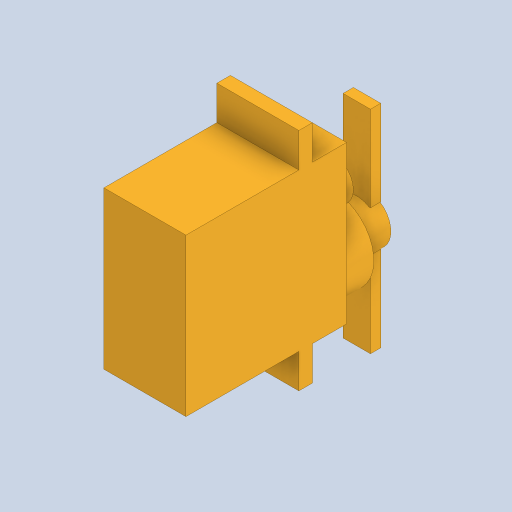
# Autodesk Inventor part: Servo
Saved by Autodesk Inventor 2023.1 (Build 271208000, 208)
## iProperties
Created: 2024-08-02
Part Number: Servo
Material: S355J2+N
Document SubType Name: Modeling
Designer: huchonms
Engineer: thingelstade
Mass: 59.7282 g
Surface Area: 30.452 cm^2
Volume: 7.60868 cm^3
Density: 7.85 g/cm^3
Appearance: Metal (300-500 MPa)
tc_part_rev_length: 12
tc_part_rev_width: 32.5
tc_part_rev_height: 37.54
tc_part_rev_uom_length: mm
tc_part_rev_volume: 7609
tc_part_rev_uom_volume: mm^3
tc_part_rev_mass: 0.06
tc_part_rev_uom_mass: kg
NOV_FileName: Servo
Author: huchonms
Revision Number: 0
Autodesk Inventor part; units mm, degrees
ref_plane "YZ Plane" through (0, 0, 0) normal (1, 0, 0) x (0, 1, 0)
ref_plane "XZ Plane" through (0, 0, 0) normal (0, 1, 0) x (-1, 0, 0)
ref_plane "XY Plane" through (0, 0, 0) normal (0, 0, 1) x (1, 0, 0)
sketch "Sketch1" plane through (0, 0, 0) normal (0, 1, 0) x (-1, 0, 0)
  line L0 (-6, -11.5) -> (6, -11.5)
  line L1 (6, -11.5) -> (6, 11.5)
  line L2 (6, 11.5) -> (-6, 11.5)
  line L3 (-6, 11.5) -> (-6, -11.5)
  line L4 (-6, -11.5) -> (6, 11.5) construction
  line L5 (6, -11.5) -> (-6, 11.5) construction
  point P0 (0, 0)
  dimension "d0" = 12
  dimension "d1" = 23
  constraints: 12 end point, 2 midpoint, 2 parallel, 1 horizontal, 1 perpendicular
  measures "d0" distance of L2.end L1.end
  measures "d1" distance of L1.end L0.end
extrude "Extrusion1" add sketch "Sketch1" along normal blind 23.5
sketch "Sketch2" plane through (-6, 0, -11.5) normal (-1, 0, 0) x (0, 0, 1)
  line L0 (0, 23.5) -> (23, 23.5) projected
  line L1 (0, 18.5) -> (23, 18.5)
  line L2 (0, 18.5) -> (0, 16.523)
  line L3 (0, 16.523) -> (23, 16.523)
  line L4 (23, 16.523) -> (23, 18.5)
  point P0 (11.5, 0)
  dimension "d7" = 5
  constraints: 8 end point, 2 perpendicular, 1 horizontal, 1 vertical
  measures "d7" distance between parallel lines of L1 L0
extrude "Extrusion2" add sketch "Sketch2" along normal blind 5
sketch "Sketch3" plane through (6, 0, 11.5) normal (1, 0, 0) x (0, 0, -1)
  line L0 (0, 16.523) -> (0, 18.5) projected
  line L1 (0, 18.5) -> (23, 18.5) projected
  line L2 (23, 18.5) -> (23, 16.523) projected
  line L3 (23, 16.523) -> (0, 16.523) projected
  point P0 (11.5, 0)
extrude "Extrusion3" add sketch "Sketch3" along normal blind 5
sketch "Sketch4" plane through (0, 23.5, 0) normal (0, 1, 0) x (1, 0, 0)
  circle A0 centre (0, 5.5) radius 6
  line L0 (6, 11.5) -> (-6, 11.5) projected
  point P0 (0, 0)
  dimension "d12" = 12
  dimension "d13" = 6
  constraints: 1 centre point
  measures "d12" diameter of A0
  measures "d13" distance from line of L0 A0.centre
extrude "Extrusion4" add sketch "Sketch4" along normal blind 4
sketch "Sketch6" plane through (0, 23.5, 0) normal (0, 1, 0) x (1, 0, 0)
  circle A0 centre (0, -2) radius 3
  point P0 (0, 0)
  dimension "d17" = 6
  constraints: 1 centre point
  measures "d17" diameter of A0
extrude "Extrusion5" add sketch "Sketch6" along normal up to surface (4 mm away)
sketch "Sketch7" plane through (-6, 0, 11.5) normal (0, 0, 1) x (1, 0, 0)
  line L0 (12, 18.5) -> (17, 18.5) projected
  line L1 (0, 18.5) -> (-5, 18.5) projected
  line L2 (0, 16.523) -> (-5, 16.523) projected
  line L3 (12, 16.523) -> (17, 16.523) projected
  line L4 (0, 18.5) -> (0, 16.523)
  line L5 (0, 16.523) -> (12, 16.523)
  line L6 (12, 16.523) -> (12, 18.5)
  line L7 (0, 18.5) -> (12, 18.5)
  point P0 (6, 0)
  constraints: 8 end point, 2 perpendicular, 1 horizontal, 1 vertical
extrude "Extrusion6" add sketch "Sketch7" along normal blind 5
sketch "Sketch8" plane through (6, 0, -11.5) normal (0, 0, -1) x (-1, 0, 0)
  line L0 (0, 18.5) -> (12, 18.5) projected
  line L1 (12, 18.5) -> (12, 16.523) projected
  line L2 (12, 16.523) -> (0, 16.523) projected
  line L3 (0, 16.523) -> (0, 18.5) projected
  point P0 (6, 0)
extrude "Extrusion7" add sketch "Sketch8" along normal blind 5
sketch "Sketch9" plane through (11, 0, 11.5) normal (1, 0, 0) x (0, 0, -1)
  line L0 (23, 16.523) -> (23, 18.5) projected
  line L1 (23, 18.5) -> (0, 18.5) projected
  line L2 (0, 18.5) -> (0, 16.523) projected
  line L3 (0, 16.523) -> (23, 16.523) projected
  point P0 (11.5, 0)
extrude "Extrusion8" cut sketch "Sketch9" against normal up to surface (5 mm away)
sketch "Sketch10" plane through (-11, 0, -11.5) normal (-1, 0, 0) x (0, 0, 1)
  line L0 (23, 16.523) -> (23, 18.5) projected
  line L1 (23, 18.5) -> (0, 18.5) projected
  line L2 (0, 18.5) -> (0, 16.523) projected
  line L3 (0, 16.523) -> (23, 16.523) projected
  point P0 (11.5, 0)
extrude "Extrusion9" cut sketch "Sketch10" against normal up to surface (5 mm away)
sketch "Sketch11" plane through (0, 27.5, 0) normal (0, 1, 0) x (1, 0, 0)
  circle A0 centre (0, 5.5352) radius 3.5
  point P0 (0, 0)
  dimension "d28" = 7
  constraints: 1 centre point
  measures "d28" diameter of A0
extrude "Extrusion10" add sketch "Sketch11" along normal blind 5
sketch "Sketch14" plane through (0, 32.5, -5.5352) normal (0, 1, 0) x (1, 0, 0)
  line L0 (-2, -3) -> (2, -3)
  line L1 (2, -3) -> (2, -15.5)
  line L2 (2, -15.5) -> (-2, -15.5)
  line L3 (-2, -15.5) -> (-2, -3)
  line L4 (-2, 3) -> (2, 3)
  line L5 (2, 3) -> (2, 15.5)
  line L6 (2, 15.5) -> (-2, 15.5)
  line L7 (-2, 15.5) -> (-2, 3)
  point P0 (0, -5.5352)
  dimension "d39" = 12.5
  dimension "d40" = 12.5
  constraints: 16 end point, 4 parallel, 2 horizontal, 2 perpendicular
  measures "d39" distance of L0.end L1.end
  measures "d40" distance of L5.end L4.end
extrude "Extrusion13" add sketch "Sketch14" against normal blind 1.5
body "Solid1"
